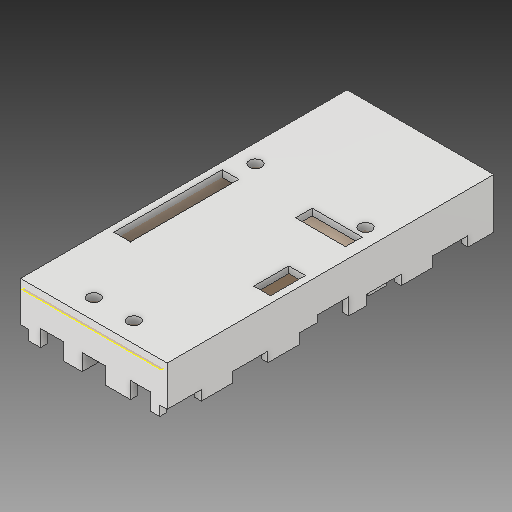
# Autodesk Inventor part: B7
Saved by Autodesk Inventor 2019.4 (Build 234330000, 330)
## iProperties
Created: 2019-05-27
Part Number: B7
Material: ABS Plastic
Document SubType Name: Modeling
Designer: Yichen Wang
Density: 1.06 g/cm^3
Appearance: Smooth - White
Mass: 15.4712 g
Surface Area: 163.292 cm^2
Volume: 14.5955 cm^3
Description: VESC CASE COVER
Author: Yichen Wang
Title: ESC CASE TOP
Autodesk Inventor part; units mm, degrees
ref_plane "YZ Plane" through (0, 0, 0) normal (1, 0, 0) x (0, 1, 0)
ref_plane "XY Plane" through (0, 0, 0) normal (0, 0, 1) x (1, 0, 0)
sketch "Sketch1" plane through (0, 0, 0) normal (0, 1, 0) x (-1, 0, 0)
  line L0 (6, 28.5) -> (-6, 28.5) construction
  line L1 (16.5, -30.5) -> (-16.5, -30.5) construction
  circle A0 centre (6, 28.5) radius 2.5
  circle A1 centre (-6, 28.5) radius 2.5
  circle A2 centre (16.5, -30.5) radius 2.5
  circle A3 centre (-16.5, -30.5) radius 2.5
  line L2 (0, 28.5) -> (0, -30.5) construction
  point P0 (0, 0)
  point P1 (0, 0)
  point P2 (0, -1)
  dimension "d2" = 12
  dimension "d3" = 33
  dimension "d5" = 5
  dimension "d55" = 1
  dimension "d56" = 59
  constraints: 6 end point, 5 coincident, 4 centre point, 3 equal radius, 3 midpoint, 2 horizontal, 1 point on line, 1 vertical
  measures "d2" distance of L0.start L0.end
  measures "d3" distance of L1.start L1.end
  measures "d5" diameter of A0
  measures "d55" distance of point (0, 0) point (0, -1)
  measures "d56" distance of L2.start L2.end
ref_plane "Work Plane1" through (0, 13, 0) normal (0, 1, 0) x (-1, 0, 0)
sketch "Sketch2" plane through (0, 13, 0) normal (0, 1, 0) x (-1, 0, 0)
  line L0 (20, 32.5) -> (8.5, 32.5)
  line L1 (-20, 32.5) -> (-20, -28)
  line L2 (-20, -32.5) -> (-14, -32.5) construction
  line L3 (20, -32.5) -> (20, -28) construction
  line L4 (20, 32.5) -> (-20, -32.5) construction
  line L5 (-20, 32.5) -> (20, -32.5) construction
  line L6 (-21, 33.5) -> (21, 33.5)
  line L7 (21, 33.5) -> (21, -33.5)
  line L8 (21, -33.5) -> (-21, -33.5)
  line L9 (-21, -33.5) -> (-21, 33.5)
  circle A0 centre (-16.5, -30.5) radius 1.5
  arc A1 (-14, -30.5) -> (-16.5, -28) centre (-16.5, -30.5) ccw
  line L10 (-14, -30.5) -> (-14, -32.5)
  line L11 (-16.5, -28) -> (-20, -28)
  line L12 (-20, -28) -> (-20, -32.5) construction
  line L13 (-14, -32.5) -> (14, -32.5)
  line L14 (0, 0) -> (0, -6.2237) construction
  circle A2 centre (16.5, -30.5) radius 1.5
  arc A3 (16.5, -28) -> (14, -30.5) centre (16.5, -30.5) ccw
  line L15 (14, -30.5) -> (14, -32.5)
  line L16 (16.5, -28) -> (20, -28)
  line L17 (20, -28) -> (20, 32.5)
  line L18 (14, -32.5) -> (20, -32.5) construction
  circle A4 centre (6, 28.5) radius 1.5
  line L19 (8.5, 32.5) -> (3.5, 32.5) construction
  line L20 (3.5, 32.5) -> (-3.5, 32.5)
  circle A5 centre (-6, 28.5) radius 1.5
  line L21 (-3.5, 32.5) -> (-8.5, 32.5) construction
  line L22 (-8.5, 32.5) -> (-20, 32.5)
  line L23 (8.5, 32.5) -> (8.5, 28.5)
  arc A6 (3.5, 28.5) -> (8.5, 28.5) centre (6, 28.5) ccw
  line L24 (3.5, 32.5) -> (3.5, 28.5)
  line L25 (8.5, 28.5) -> (3.5, 28.5) construction
  line L26 (-3.5, 32.5) -> (-3.5, 28.5)
  arc A7 (-8.5, 28.5) -> (-3.5, 28.5) centre (-6, 28.5) ccw
  line L27 (-8.5, 28.5) -> (-8.5, 32.5)
  dimension "d9" = 40
  dimension "d10" = 65
  dimension "d11" = 1
  dimension "d14" = 3
  dimension "d15" = 2.5
  dimension "d16" = 1
  dimension "d17" = 1
  dimension "d18" = 1
  dimension "d19" = 3
  dimension "d23" = 2.5
  dimension "d24" = 2.5
  constraints: 56 end point, 21 parallel, 16 perpendicular, 9 point on circle, 9 symmetric about line, 8 centre point, 7 coincident, 6 horizontal, 5 vertical, 3 midpoint, 3 tangent, 1 point on line, 3 other
  measures "d9" distance of L3.start L2.start
  measures "d10" distance of L2.start L1.start
  measures "d11" distance between parallel lines of L0 L6
  measures "d14" diameter of A0
  measures "d15" radius of A1
  measures "d16" distance between parallel lines of L13 L8
  measures "d17" distance between parallel lines of L1 L9
  measures "d18" distance between parallel lines of L17 L7
  measures "d19" diameter of A4
  measures "d23" radius of A6
  measures "d24" radius of A7
extrude "Extrusion3" add sketch "Sketch2" against normal blind 13
sketch "Sketch3" plane through (0, 13, 0) normal (0, 1, 0) x (-1, 0, 0)
  line L0 (-21, 33.5) -> (21, 33.5) projected
  line L1 (-21, -33.5) -> (-21, 33.5) projected
  line L2 (21, 33.5) -> (-21, 33.5)
  line L3 (-21, 33.5) -> (-21, -33.5)
  line L4 (-21, -33.5) -> (21, -33.5)
  line L5 (21, -33.5) -> (21, 33.5)
  point P0 (0, 0)
  constraints: 8 end point, 2 parallel, 1 horizontal, 1 perpendicular
extrude "Extrusion4" add sketch "Sketch3" along normal blind 1
sketch "Sketch4" plane through (-21, 0, 33.5) normal (0, 0, 1) x (1, 0, 0)
  line L0 (12, -5) -> (5, -5)
  line L1 (5, -5) -> (5, 5)
  line L2 (5, 5) -> (12, 5)
  line L3 (12, 5) -> (12, -5)
  line L4 (42, 0) -> (0, 0) projected
  line L5 (12, -5) -> (5, 5) construction
  line L6 (5, -5) -> (12, 5) construction
  line L7 (24.5, -5) -> (17.5, -5)
  line L8 (17.5, -5) -> (17.5, 5)
  line L9 (17.5, 5) -> (24.5, 5)
  line L10 (24.5, 5) -> (24.5, -5)
  line L11 (24.5, -5) -> (17.5, 5) construction
  line L12 (17.5, -5) -> (24.5, 5) construction
  line L13 (38, -5) -> (32, -5)
  line L14 (32, -5) -> (32, 5)
  line L15 (32, 5) -> (38, 5)
  line L16 (38, 5) -> (38, -5)
  line L17 (38, -5) -> (32, 5) construction
  line L18 (32, -5) -> (38, 5) construction
  point P0 (21, 0)
  point P1 (8.5, 0)
  point P2 (35, 0)
  dimension "d29" = 10
  dimension "d30" = 10
  dimension "d31" = 7
  dimension "d32" = 7
  dimension "d33" = 6
  dimension "d34" = 4
  dimension "d35" = 5
  constraints: 36 end point, 6 midpoint, 6 parallel, 3 horizontal, 3 perpendicular, 3 point on line
  measures "d29" distance of L2.end L0.start
  measures "d30" distance of L7.end L8.end
  measures "d31" distance of L1.end L2.end
  measures "d32" distance of L8.end L9.end
  measures "d33" distance of L14.end L15.end
  measures "d34" distance from line of L4.start L16
  measures "d35" distance from line of L4.end L1
extrude "Extrusion5" cut sketch "Sketch4" against normal up to surface (1 mm away)
sketch "Sketch6" plane through (21, 0, -33.5) normal (0, 0, -1) x (-1, 0, 0)
  line L0 (42, 0) -> (0, 0) projected
  line L1 (42, 14) -> (42, 0) projected
  line L2 (0, 0) -> (42, 0)
  line L3 (42, 0) -> (42, 14)
  line L4 (42, 14) -> (0, 14)
  line L5 (0, 14) -> (0, 0)
  line L6 (1, 0) -> (41, 0)
  line L7 (41, 0) -> (41, 13)
  line L8 (41, 13) -> (1, 13)
  line L9 (1, 13) -> (1, 0)
  point P0 (21, 0)
  dimension "d43" = 1
  dimension "d44" = 1
  dimension "d45" = 1
  constraints: 16 end point, 4 parallel, 2 horizontal, 2 perpendicular, 1 point on line
  measures "d43" distance between parallel lines of L1 L7
  measures "d44" distance between parallel lines of L4 L8
  measures "d45" distance between parallel lines of L5 L9
extrude "Extrusion7" add sketch "Sketch6" along normal blind 30 contours L0 L7 L8 L9 L5 L4 L1
hole "Hole1" at (-16.5, 0, -30.5) at (16.5, 0, -30.5) at (6, 0, 28.5) at (-6, 0, 28.5) direction (0, 1, 0) diameter 3.7 end through all both
sketch "Sketch7" plane through (0, 0, 0) normal (0, -1, 0) x (1, 0, 0)
  line L0 (-21, 33.5) -> (-21, -63.5) projected
  line L1 (-21, 33.5) -> (-20, 33.5)
  line L2 (-20, 33.5) -> (-20, 24.25)
  line L3 (-20, 24.25) -> (-21, 24.25)
  line L4 (-21, 24.25) -> (-21, 33.5)
  line L5 (-20, 14.75) -> (-21, 14.75)
  line L6 (-21, 14.75) -> (-21, 4.25)
  line L7 (-21, 4.25) -> (-20, 4.25)
  line L8 (-20, 4.25) -> (-20, 14.75)
  line L9 (-21, -5.25) -> (-20, -5.25)
  line L10 (-20, -5.25) -> (-20, -15.75)
  line L11 (-20, -15.75) -> (-21, -15.75)
  line L12 (-21, -15.75) -> (-21, -5.25)
  line L13 (-21, -25.25) -> (-20, -25.25)
  line L14 (-20, -25.25) -> (-20, -35.75)
  line L15 (-20, -35.75) -> (-21, -35.75)
  line L16 (-21, -35.75) -> (-21, -25.25)
  line L17 (-20, -45.25) -> (-21, -45.25)
  line L18 (-21, -45.25) -> (-21, -55.75)
  line L19 (-21, -55.75) -> (-20, -55.75)
  line L20 (-20, -55.75) -> (-20, -45.25)
  point P0 (0, 0)
  dimension "d81" = 1
  dimension "d82" = 9.25
  dimension "d83" = 9.5
  dimension "d84" = 10.5
  dimension "d85" = 9.5
  dimension "d86" = 10.5
  dimension "d87" = 9.5
  dimension "d88" = 10.5
  dimension "d89" = 9.5
  dimension "d90" = 10.5
  constraints: 40 end point, 10 parallel, 7 point on line, 5 horizontal, 5 perpendicular, 1 collinear
  measures "d81" distance of L0.start L1.end
  measures "d82" distance of L1.end L2.end
  measures "d83" distance between parallel lines of L5 L3
  measures "d84" distance of L7.end L5.start
  measures "d85" distance between parallel lines of L9 L7
  measures "d86" distance of L9.end L10.end
  measures "d87" distance between parallel lines of L13 L11
  measures "d88" distance of L13.end L14.end
  measures "d89" distance between parallel lines of L17 L15
  measures "d90" distance of L19.end L17.start
extrude "Extrusion8" cut sketch "Sketch7" against normal blind 3
mirror "Mirror1" about plane through (0, 0, 0) normal (1, 0, 0) of "Extrusion8"
sketch "Sketch5" plane through (21, 0, 33.5) normal (1, 0, 0) x (0, 0, -1)
  line L0 (61.5, 0) -> (1, 0) projected
  line L1 (44, 0) -> (53, 0)
  line L2 (53, 0) -> (53, 5)
  line L3 (53, 5) -> (44, 5)
  line L4 (44, 5) -> (44, 0)
  line L5 (67, 14) -> (67, 0) projected
  line L6 (44, 0) -> (53, 0)
  line L7 (53, 0) -> (53, -11.8945)
  line L8 (53, -11.8945) -> (44, -11.8945)
  line L9 (44, -11.8945) -> (44, 0)
  point P0 (33.5, 0)
  dimension "d38" = 5
  dimension "d39" = 9
  dimension "d40" = 14
  constraints: 16 end point, 4 parallel, 2 horizontal, 2 perpendicular, 1 point on line
  measures "d38" distance of L3.end L1.start
  measures "d39" distance of L2.end L3.end
  measures "d40" distance between parallel lines of L5 L2
extrude "Extrusion6" cut sketch "Sketch5" against normal up to surface (1 mm away)
thicken "Thicken2" operation add thickness 1 both sides no extend neighbours yes toward (-1, 0, 0) faces at (-21, 10.3333, -11.75) (1.1667, 11, 33.5) (21, 11, -13.5) (-1.8524, 14, -10.34)
thicken "Thicken3" operation add thickness 0.25 both sides no extend neighbours yes toward (-1, 0, 0) faces at (20, 2, 33.1667)
thicken "Thicken4" operation add thickness 0.25 both sides no extend neighbours yes toward (1, 0, 0) faces at (-20, 2, 33.1667)
thicken "Thicken5" operation add thickness 0.25 both sides no extend neighbours yes toward (-1, 0, 0) faces at (20, 2, -31.6667)
thicken "Thicken6" operation add thickness 0.25 both sides no extend neighbours yes toward (1, 0, 0) faces at (-20, 1, -29.8333)
thicken "Thicken7" operation add thickness 0.5 both sides no extend neighbours yes toward (0, 0, -1) faces at (21.3333, 1.6667, -19.5)
sketch "Sketch8" plane through (0, 13, 0) normal (0, -1, 0) x (1, 0, 0)
  line L0 (-20, 32.5) -> (-20, -28) projected
  line L1 (-20, 8.5) -> (-15, 8.5)
  line L2 (-15, 8.5) -> (-15, -24)
  line L3 (-15, -24) -> (-20, -24)
  line L4 (-20, -24) -> (-20, 8.5)
  line L5 (-19.75, 32.5) -> (-16, 32.5) projected
  circle A0 centre (-16.5, -30.5) radius 1.85 projected
  line L6 (3.5, -27.5) -> (18.5, -27.5)
  line L7 (18.5, -27.5) -> (18.5, -22.5)
  line L8 (18.5, -22.5) -> (3.5, -22.5)
  line L9 (3.5, -22.5) -> (3.5, -27.5)
  line L10 (20, -28) -> (20, -25.25) projected
  circle A1 centre (16.5, -30.5) radius 1.85 projected
  line L11 (20, -28) -> (20, 32.5) projected
  line L12 (20, -9) -> (15, -9)
  line L13 (15, -9) -> (15, 1.5)
  line L14 (15, 1.5) -> (20, 1.5)
  line L15 (20, 1.5) -> (20, -9)
  line L16 (17, 32.5) -> (19.75, 32.5) projected
  point P0 (0, 0)
  dimension "d103" = 24
  dimension "d104" = 6.5
  dimension "d105" = 5
  dimension "d106" = 1.5
  dimension "d107" = 15
  dimension "d108" = 3
  dimension "d109" = 5
  dimension "d110" = 31
  dimension "d111" = 10.5
  dimension "d112" = 5
  constraints: 24 end point, 6 parallel, 3 horizontal, 3 perpendicular, 2 point on line
  measures "d103" distance between parallel lines of L5 L1
  measures "d104" distance from line of A0.centre L3
  measures "d105" distance of L1.start L1.end
  measures "d106" distance between parallel lines of L10 L7
  measures "d107" distance of L7.end L8.end
  measures "d108" distance from line of L6 A1.centre
  measures "d109" distance of L8.end L6.start
  measures "d110" distance between parallel lines of L16 L14
  measures "d111" distance of L12.end L13.end
  measures "d112" distance of L13.end L14.end
extrude "Extrusion9" cut sketch "Sketch8" against normal blind 10 contours L1 L2 L3 L0 | L9 L8 L7 L6 | L12 L13 L14 L11
equation "\"d85\" = d83"
equation "\"d86\" = d84"
equation "\"d87\" = d83"
equation "\"d88\" = d84"
equation "\"d89\" = d83"
equation "\"d90\" = d84"
body "Solid3"
